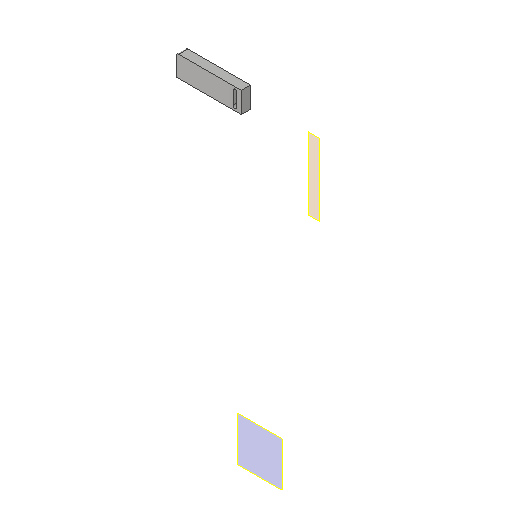
# Autodesk Inventor part: 20_Cube_Insert_Beamsplittercube_motorized_gearmount
Saved by Autodesk Inventor 2022 (Build 260153000, 153)
## iProperties
Created: 2021-10-11
Part Number: 20_Cube_Insert_Beamsplittercube_motorized_gearmount
Material: Generic
Document SubType Name: Modeling
Designer: diederichbenedict
Density: 1 g/cm^3
Appearance: Default
Author: diederichbenedict
Autodesk Inventor part; units mm, degrees
ref_plane "YZ Plane" through (0, 0, 0) normal (1, 0, 0) x (0, 1, 0)
ref_plane "XZ Plane" through (0, 0, 0) normal (0, 1, 0) x (-1, 0, 0)
ref_plane "XY Plane" through (0, 0, 0) normal (0, 0, 1) x (1, 0, 0)
ref_plane "Work Plane1" through (0, 0, 0) normal (0, 0, 1) x (1, 0, 0)
ref_plane "Arbeitsebene4" through (20.8809, -161.4072, 41.121) normal (0, 0, -1) x (-1, 0.0000136, 0)
sketch "Skizze2" plane through (20.8809, -161.4072, 41.121) normal (0, 0, -1) x (-1, 0.0000136, 0)
  line L0 (12.108, 248.7648) -> (12.1074, 202.9648) projected
  line L1 (61.9074, 202.9641) -> (61.908, 248.7641) projected
  line L2 (12.108, 248.7648) -> (12.1074, 202.9648) projected
  line L3 (12.1076, 217.8647) -> (61.9078, 217.8647)
  line L4 (61.9078, 217.8647) -> (61.9078, 233.8647)
  line L5 (61.9078, 233.8647) -> (12.1076, 233.8647)
  line L6 (12.1076, 233.8647) -> (12.1076, 217.8647)
  circle A0 centre (35.4547, 209.435) radius 1.4 projected
  circle A1 centre (-0.5528, 14.7177) radius 1.9
  line L7 (17.0077, 230.8647) -> (17.0077, 220.8647) construction
  line L8 (15.6077, 230.8647) -> (15.6077, 220.8647)
  line L9 (18.4077, 220.8647) -> (18.4077, 230.8647)
  arc A2 (18.4077, 230.8647) -> (15.6077, 230.8647) centre (17.0077, 230.8647) ccw
  arc A3 (15.6077, 220.8647) -> (18.4077, 220.8647) centre (17.0077, 220.8647) ccw
  line L10 (57.0077, 230.8642) -> (57.0077, 220.8642) construction
  line L11 (55.6077, 230.8642) -> (55.6077, 220.8642)
  line L12 (58.4077, 220.8642) -> (58.4077, 230.8642)
  arc A4 (58.4077, 230.8642) -> (55.6077, 230.8642) centre (57.0077, 230.8642) ccw
  arc A5 (55.6077, 220.8642) -> (58.4077, 220.8642) centre (57.0077, 220.8642) ccw
  circle A6 centre (57.0077, 225.8642) radius 1.4 projected
  circle A7 centre (17.0077, 225.8647) radius 1.4 projected
  point P0 (20.8831, 161.4069)
  point P1 (12.1078, 233.8647)
  point P2 (12.1076, 217.8647)
  point P3 (61.9076, 217.8647)
  point P4 (55.9077, 226.7302)
  point P5 (55.9077, 224.9982)
  point P6 (17.6738, 227.0961)
  point P7 (17.6738, 224.6333)
  dimension "d8" = 3.8
  constraints: 24 end point, 8 point on circle, 8 tangent, 5 centre point, 5 parallel, 2 point on line, 1 horizontal, 1 perpendicular, 1 vertical
  measures "d8" diameter of A1
extrude "Extrusion2" add sketch "Skizze2" along normal blind 5 contours L5 L1 L3 L0
fillet "Rundung1" radius 2 1 edges at (-41.0238, 72.4584, 38.621)
sketch "Skizze3" plane through (20.8809, -161.4072, 41.121) normal (0, 0, 1) x (1, -0.0000136, 0)
  line L0 (-17.6739, 230.8647) -> (-17.6738, 227.0961) projected
  line L1 (-12.1076, 217.8647) -> (-61.9078, 217.8647) projected
  arc A0 (-59.9078, 233.8647) -> (-61.9078, 231.8647) centre (-59.9078, 231.8647) ccw projected
  line L2 (-59.9078, 233.8647) -> (-12.1076, 233.8647) projected
  arc A1 (-15.6077, 230.8647) -> (-18.4077, 230.8647) centre (-17.0077, 230.8647) ccw projected
  line L3 (-18.4077, 230.8647) -> (-18.4077, 220.8647) projected
  arc A2 (-18.4077, 220.8647) -> (-15.6077, 220.8647) centre (-17.0077, 220.8647) ccw projected
  line L4 (-15.6077, 220.8647) -> (-15.6077, 230.8647) projected
  line L5 (-54.058, 242.9142) -> (-54.0575, 208.8142) projected
  line L6 (-12.1076, 217.8647) -> (-61.9078, 217.8647) projected
  line L7 (-54.0576, 217.8647) -> (-54.0578, 233.8647)
  line L8 (16.9671, 217.8647) -> (16.9669, 233.8647)
  line L9 (-59.9078, 233.8647) -> (-12.1076, 233.8647) projected
  line L10 (-12.1076, 233.8647) -> (-12.1076, 217.8647) projected
  line L11 (-61.9078, 217.8647) -> (-61.9078, 231.8647) projected
  point P0 (-20.8831, 161.4069)
  point P1 (21.9, 20.5542)
  point P2 (21.9, 4.5542)
  point P3 (-23.9, 4.5542)
  point P4 (15.968, 203.0968)
  point P5 (15.9675, 187.0968)
  point P6 (-54.0576, 217.8647)
  constraints: 4 end point, 3 point on line, 1 parallel, 5 other
extrude "Extrusion3" add sketch "Skizze3" along normal blind 2
equation "\"d9\" = d11"
equation "\"d11\" = 5"
